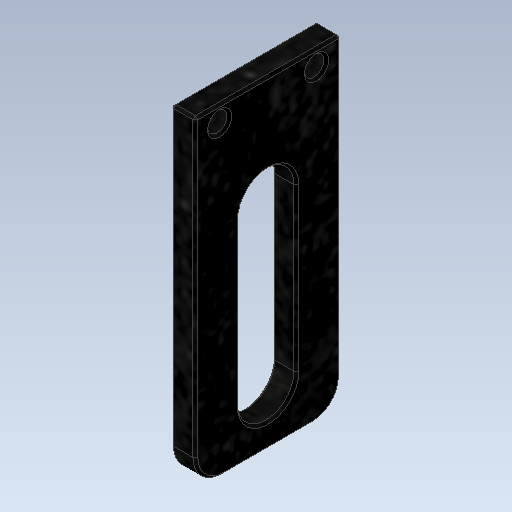
# Autodesk Inventor part: Ramka2
Saved by Autodesk Inventor 2020 (Build 240168000, 168)
## iProperties
Created: 2020-08-21
Part Number: Ramka2
Material: Steel(1)
Document SubType Name: Modeling
Designer: estee
Density: 7.85 g/cm^3
Appearance: Plate(1)
Author: estee
Autodesk Inventor part; units mm, degrees
ref_plane "YZ Plane" through (0, 0, 0) normal (1, 0, 0) x (0, 1, 0)
ref_plane "XZ Plane" through (0, 0, 0) normal (0, 1, 0) x (-1, 0, 0)
ref_plane "XY Plane" through (0, 0, 0) normal (0, 0, 1) x (1, 0, 0)
sketch "Sketch1" plane through (0, 0, 0) normal (1, 0, 0) x (0, 1, 0)
  line L0 (0, 0) -> (-36.5, 0)
  line L1 (-40, -3.5) -> (-40, -14.5)
  line L2 (-36.5, -18) -> (0, -18)
  line L3 (0, -18) -> (0, 0)
  line L4 (-13.5, -5.5) -> (-33.5, -5.5)
  line L5 (-37, -9) -> (-37, -9)
  line L6 (-33.5, -12.5) -> (-13.5, -12.5)
  line L7 (-10, -9) -> (-10, -9)
  arc A0 (-37, -9) -> (-33.5, -12.5) centre (-33.5, -9) ccw
  arc A1 (-33.5, -5.5) -> (-37, -9) centre (-33.5, -9) ccw
  arc A2 (-10, -9) -> (-13.5, -5.5) centre (-13.5, -9) ccw
  arc A3 (-13.5, -12.5) -> (-10, -9) centre (-13.5, -9) ccw
  arc A4 (-36.5, 0) -> (-40, -3.5) centre (-36.5, -3.5) ccw
  arc A5 (-40, -14.5) -> (-36.5, -18) centre (-36.5, -14.5) ccw
  point P0 (-40, -18)
  point P1 (-10, -5.5)
  point P2 (-37, -12.5)
  point P3 (-10, -12.5)
  dimension "d0" = 40
  dimension "d1" = 18
  dimension "d2" = 27
  dimension "d3" = 7
  dimension "d4" = 5.5
  dimension "d5" = 10
  dimension "d6" = 3.5
  constraints: 16 end point, 12 point on circle, 12 tangent, 8 point on line, 6 centre point, 5 equal radius, 4 parallel, 2 horizontal, 2 perpendicular
  measures "d0" distance of L2.end point (-40, -18)
  measures "d1" distance of L2.end L0.start
  measures "d2" distance of point (-10, -12.5) point (-37, -12.5)
  measures "d3" distance of point (-10, -12.5) point (-10, -5.5)
  measures "d4" distance between parallel lines of L0 L4
  measures "d5" distance between parallel lines of L3 L7
  measures "d6" radius of A0
extrude "Extrusion1" add sketch "Sketch1" along normal blind 3
sketch "Sketch2" plane through (3, 0, 0) normal (1, 0, 0) x (0, 0, -1)
  line L0 (18, 0) -> (0, 0) projected
  line L1 (0, 0) -> (0, -36.5) projected
  line L2 (18, -36.5) -> (18, 0) projected
  point P0 (3, -2)
  point P1 (15, -2)
  dimension "d9" = 2
  dimension "d10" = 2
  dimension "d11" = 3
  dimension "d12" = 3
  measures "d9" distance from line of L0 point (3, -2)
  measures "d10" distance from line of L0 point (15, -2)
  measures "d11" distance from line of L1 point (3, -2)
  measures "d12" distance from line of L2 point (15, -2)
hole "Hole1" at (3, -2, -3) at (3, -2, -15) direction (-1, 0, 0) diameter 2.4 depth 8.8 tip angle 118
chamfer "Chamfer1" distance 0.3 angle 45 26 edges at (0, 0, -9) (3, 0, -9) (1.5, 0, 0) (3, -18.25, 0) (3, -38.9749, -1.0251) (3, -40, -9) (3, -38.9749, -16.9749) (3, -18.25, -18) (0, -18.25, 0) (0, -38.9749, -1.0251) (0, -40, -9) (0, -38.9749, -16.9749) (0, -18.25, -18) (3, -2, -13.8) (3, -2, -1.8) (3, -10, -9) (3, -23.5, -12.5) (3, -37, -9) (3, -23.5, -5.5) (0, -23.5, -12.5) (0, -10, -9) (0, -23.5, -5.5) (0, -37, -9) (1.5, 0, -18) (0, -2, -13.8) (0, -2, -1.8)
body "Solid1"
